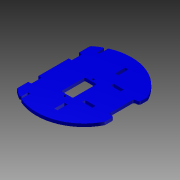
# Autodesk Inventor part: OpenROV 2.3 Dev EChassis Servo Plate
Saved by Autodesk Inventor 2012 (Build 160160000, 160)
## iProperties
Created: 2011-12-20
Part Number: OpenROV 2.3 Dev EChassis Servo Plate
Document SubType Name: Modeling
Designer: user
Density: 1 g/cm^3
Material: Default
Author: user
Autodesk Inventor part; units mm, degrees
ref_plane "YZ Plane" through (0, 0, 0) normal (1, 0, 0) x (0, 1, 0)
ref_plane "XZ Plane" through (0, 0, 0) normal (0, 1, 0) x (-1, 0, 0)
ref_plane "XY Plane" through (0, 0, 0) normal (0, 0, 1) x (1, 0, 0)
sketch "Sketch1" plane through (0, 0, 0) normal (0, 0, 1) x (1, 0, 0)
  line L0 (5.75, 25.008) -> (8.75, 25.008)
  line L1 (8.75, 35.008) -> (5.75, 35.008)
  line L2 (5.75, 35.008) -> (5.75, 25.008)
  line L3 (5.75, -24.992) -> (8.75, -24.992)
  line L4 (8.75, -34.992) -> (5.75, -34.992)
  line L5 (5.75, -34.992) -> (5.75, -24.992)
  line L6 (-4.75, 6.7) -> (4.75, 6.7)
  line L7 (5.75, 5.7) -> (5.75, -15.8)
  line L8 (4.75, -16.8) -> (-4.75, -16.8)
  line L9 (-5.75, -15.8) -> (-5.75, 5.7)
  circle A0 centre (-0.025, 9.2) radius 1.1
  circle A1 centre (-0.025, -19.3) radius 1.1
  arc A2 (-4.75, 6.7) -> (-5.75, 5.7) centre (-4.75, 5.7) ccw
  arc A3 (5.75, 5.7) -> (4.75, 6.7) centre (4.75, 5.7) ccw
  arc A4 (4.75, -16.8) -> (5.75, -15.8) centre (4.75, -15.8) ccw
  arc A5 (-5.75, -15.8) -> (-4.75, -16.8) centre (-4.75, -15.8) ccw
  line L10 (8.75, -34.992) -> (8.75, -24.992)
  line L11 (8.75, 25.008) -> (8.75, 35.008)
  line L12 (13.75, -15.5) -> (23.75, -15.5)
  line L13 (23.75, -15.5) -> (23.75, -12.5)
  line L14 (23.75, -12.5) -> (13.75, -12.5)
  line L15 (13.75, -12.5) -> (13.75, -15.5)
  line L16 (13.75, 12.5) -> (23.75, 12.5)
  line L17 (23.75, 12.5) -> (23.75, 15.5)
  line L18 (23.75, 15.5) -> (13.75, 15.5)
  line L19 (13.75, 15.5) -> (13.75, 12.5)
  line L20 (40, -12.5) -> (39, -12.5)
  line L21 (37, -10.5) -> (37, 10.5)
  line L22 (39, 12.5) -> (40, 12.5)
  arc A6 (42, -14.5) -> (40, -12.5) centre (40, -14.5) ccw
  arc A7 (37, -10.5) -> (39, -12.5) centre (39, -10.5) ccw
  arc A8 (39, 12.5) -> (37, 10.5) centre (39, 10.5) ccw
  arc A9 (40, 12.5) -> (42, 14.5) centre (40, 14.5) ccw
  line L23 (42, 14.5) -> (42, 20.6155)
  line L24 (42, -14.5) -> (42, -20.6155)
  arc A10 (41.7778, -21.5318) -> (42, -20.6155) centre (40, -20.6155) ccw
  arc A11 (42, 20.6155) -> (41.7778, 21.5318) centre (40, 20.6155) ccw
  line L25 (-30, 25) -> (-27, 25)
  line L26 (-27, 25) -> (-27, 15)
  line L27 (-27, 15) -> (-30, 15)
  line L28 (-30, -15) -> (-27, -15)
  line L29 (-27, -15) -> (-27, -25)
  line L30 (-27, -25) -> (-30, -25)
  line L31 (-32, 25.008) -> (-32, 25)
  line L32 (-32, -25) -> (-32, -24.992)
  line L33 (-30, 15) -> (-30, -15)
  arc A12 (-31.3765, -34.992) -> (-31.3333, -35.0317) centre (-30, -33.541) ccw
  arc A13 (-21, 35) -> (-19, 35) centre (-20, 35) ccw
  line L34 (-21, 35) -> (-21, 40.398)
  line L35 (-19, 35) -> (-19, 42.332)
  arc A14 (41.7778, 21.5318) -> (-18.3913, 43.2523) centre (0, 0) ccw
  arc A15 (-22.4783, 41.2762) -> (-29.2444, 36.7935) centre (0, 0) ccw
  arc A16 (-19, -35) -> (-21, -35) centre (-20, -35) ccw
  line L36 (-21, -35) -> (-21, -40.398)
  line L37 (-19, -35) -> (-19, -42.332)
  arc A17 (-29.2444, -36.7935) -> (-22.4783, -41.2762) centre (0, 0) ccw
  arc A18 (-18.3913, -43.2523) -> (41.7778, -21.5318) centre (0, 0) ccw
  arc A19 (-22.4783, -41.2762) -> (-21, -40.398) centre (-22, -40.398) ccw
  arc A20 (-19, -42.332) -> (-18.3913, -43.2523) centre (-18, -42.332) ccw
  arc A21 (-21, 40.398) -> (-22.4783, 41.2762) centre (-22, 40.398) ccw
  arc A22 (-18.3913, 43.2523) -> (-19, 42.332) centre (-18, 42.332) ccw
  line L38 (-30, 25) -> (-30, 35.2278)
  line L39 (-30, -25) -> (-30, -35.2278)
  arc A23 (-30, -35.2278) -> (-29.2444, -36.7935) centre (-28, -35.2278) ccw
  arc A24 (-29.2444, 36.7935) -> (-30, 35.2278) centre (-28, 35.2278) ccw
  point P0 (5.75, -16.8)
  point P1 (-5.75, -16.8)
  point P2 (8.75, -46.1783)
  point P3 (37, 12.5)
  point P4 (37, -12.5)
  point P5 (42, 21.095)
  point P6 (42, -21.095)
  point P7 (-30, 36.1801)
  point P8 (-21, 42.0476)
  point P9 (-19, 42.9884)
  point P10 (-21, -42.0476)
  point P11 (-19, -42.9884)
  point P12 (-30, -36.1801)
  dimension "d13" = 10
  dimension "d17" = 10
  dimension "d51" = 11.5
  dimension "d52" = 23.5
  dimension "d54" = 2.2
  dimension "d55" = 2.5
  dimension "d56" = 2.2
  dimension "d57" = 2.5
  dimension "d58" = 1
  dimension "d69" = 0
  dimension "d70" = 3
  dimension "d71" = 0
  dimension "d72" = 3
  dimension "d113" = 10
  dimension "d114" = 3
  dimension "d115" = 10
  dimension "d116" = 3
  dimension "d117" = 25
  dimension "d119" = 5
  dimension "d122" = 5
  dimension "d125" = 25
  dimension "d126" = 2
  dimension "d131" = 5.75
  dimension "d132" = 6.7
  dimension "d133" = 2
  dimension "d136" = 10
  dimension "d137" = 10
  dimension "d140" = 15
  dimension "d141" = 15
  dimension "d143" = 2
  dimension "d145" = 10
  dimension "d146" = 47
  dimension "d147" = 47
  dimension "d149" = 2
  dimension "d150" = 10
  dimension "d152" = 1
  dimension "d153" = 30
  dimension "d154" = 27
  dimension "d155" = 32
  dimension "d156" = 27
  dimension "d157" = 2
  constraints: 80 end point, 52 point on circle, 34 tangent, 25 centre point, 19 point on line, 18 parallel, 11 equal radius, 8 horizontal, 8 perpendicular, 2 collinear
  measures "d13" distance of L1.end L0.start
  measures "d17" distance of L4.end L3.start
  measures "d51" distance of point (5.75, -16.8) point (-5.75, -16.8)
  measures "d52" distance between parallel lines of L8 L6
  measures "d54" diameter of A0
  measures "d55" distance from line of A0.centre L6
  measures "d56" diameter of A1
  measures "d57" distance from line of A1.centre L8
  measures "d58" radius of A2
  measures "d69" distance between parallel lines of L2 L7
  measures "d70" distance of L1.start L1.end
  measures "d71" distance between parallel lines of L5 L7
  measures "d72" distance of L4.start L4.end
  measures "d113" distance of L12.start L12.end
  measures "d114" distance of L14.end L12.start
  measures "d115" distance of L16.start L16.end
  measures "d116" distance of L18.end L16.start
  measures "d117" distance between parallel lines of L14 L16
  measures "d119" distance between parallel lines of L10 L15
  measures "d122" distance between parallel lines of L11 L19
  measures "d125" distance of point (37, -12.5) point (37, 12.5)
  measures "d126" radius of A6
  measures "d131" distance from line of A14.centre L9
  measures "d132" distance from line of A14.centre L6
  measures "d133" radius of A10
  measures "d136" distance of L25.end L26.end
  measures "d137" distance of L28.end L29.end
  measures "d140" distance from line of A14.centre L27
  measures "d141" distance from line of A14.centre L28
  measures "d143" diameter of A13
  measures "d145" distance from line of L25 A13.centre
  measures "d146" radius of A14
  measures "d147" radius of A15
  measures "d149" diameter of A16
  measures "d150" distance from line of A16.centre L30
  measures "d152" radius of A19
  measures "d153" distance from line of L33 A14.centre
  measures "d154" distance from line of A14.centre L26
  measures "d155" distance from line of A14.centre L31
  measures "d156" distance from line of A14.centre L29
  measures "d157" radius of A23
extrude "Extrusion8" add sketch "Sketch1" along normal blind 3
body "Solid8"
